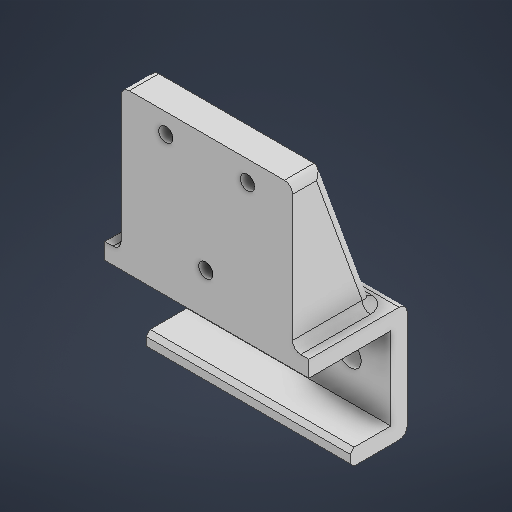
# Autodesk Inventor part: Optical Camera 8020 Bracket
Saved by Autodesk Inventor 2026.2 (Build 302298000, 298)
## iProperties
Created: 2026-02-05
Part Number: Optical Camera 8020 Bracket
Material: Generic
Document SubType Name: Modeling
Designer: mumin
Density: 1 g/cm^3
Appearance: Default
Author: mumin
Autodesk Inventor part; units mm, degrees
ref_plane "YZ Plane" through (0, 0, 0) normal (1, 0, 0) x (0, 1, 0)
ref_plane "XZ Plane" through (0, 0, 0) normal (0, 1, 0) x (-1, 0, 0)
ref_plane "XY Plane" through (0, 0, 0) normal (0, 0, 1) x (1, 0, 0)
sketch "Sketch1" plane through (0, 0, 0) normal (1, 0, 0) x (0, 1, 0)
  line L0 (0, 0) -> (0, -20.1)
  line L1 (0, -20.1) -> (-20.2, -20.1)
  line L2 (-20.2, -20.1) -> (-20.2, -10.1)
  line L3 (-20.2, -10.1) -> (-24.2, -10.1)
  line L4 (-24.2, -10.1) -> (-24.2, -22.1)
  line L5 (-22.2, -24.1) -> (2, -24.1)
  line L6 (4, -22.1) -> (4, 0)
  line L7 (4, 0) -> (0, 0)
  arc A0 (-24.2, -22.1) -> (-22.2, -24.1) centre (-22.2, -22.1) ccw
  arc A1 (2, -24.1) -> (4, -22.1) centre (2, -22.1) ccw
  line L8 (4, 0) -> (39, 0)
  line L9 (39, 0) -> (39, -7.25)
  line L10 (39, -7.25) -> (4, -7.25)
  dimension "d0" = 20.1
  dimension "d1" = 20.2
  dimension "d2" = 10
  dimension "d3" = 4
  dimension "d4" = 4
  dimension "d5" = 4
  dimension "d7" = 35
  dimension "d8" = 7.25
  constraints: 22 end point, 9 perpendicular, 4 point on circle, 4 tangent, 2 centre point, 1 horizontal, 1 point on line, 1 vertical
  measures "d0" distance of L0.start L0.end
  measures "d1" distance of L0.end L1.end
  measures "d2" distance of L1.end L2.end
  measures "d3" distance of L3.end L2.end
  measures "d4" distance between parallel lines of L5 L1
  measures "d5" distance between parallel lines of L0 L6
  measures "d7" distance of L6.end L8.end
  measures "d8" distance of L8.end L9.end
extrude "Beam Clip" add sketch "Sketch1" along normal mid plane 50 contours L7 L6 A1 L5 A0 L4 L3 L2 L1 L0
extrude "Camera Mount Face" add sketch "Sketch1" along normal mid plane 32 contours L8 L9 L10 L6
sketch "Sketch2" plane through (16, 39, -7.25) normal (0, 0, -1) x (-1, 0, 0)
  line L0 (16.0101, -1.1873) -> (16.2932, -34.4018)
  line L1 (32, 0) -> (0, 0) projected
  point P0 (16, -39)
  point P1 (16, 0)
  point P2 (16.2446, -28.7)
  point P3 (6.0422, -5)
  point P4 (26.0415, -4.8296)
  dimension "d14" = 20
  dimension "d38" = 5
  dimension "d39" = 23.7
  constraints: 2 end point, 2 point on line, 1 midpoint, 1 symmetric about line
  measures "d14" diameter of point (6.042, -5) L0
  measures "d38" distance from line of L1 point (6.042, -5)
  measures "d39" vertical distance of point (16.245, -28.7) point (6.042, -5)
hole "Camera Mount Holes" at (-10.0415, 34.1704, -7.25) at (-0.2446, 10.3, -7.25) at (9.9578, 34, -7.25) direction (0, 0, 1) diameter 3.5 end through all
sketch "Sketch3" plane through (16, 0, 0) normal (1, 0, 0) x (0, 0, -1)
  line L0 (7.25, 4) -> (7.25, 39) projected
  line L1 (7.25, 39) -> (19.9087, 4)
  line L2 (22.1, 4) -> (0, 4) projected
  line L3 (0, 39) -> (0, 4) projected
  line L4 (0, 4) -> (0, 39)
  line L5 (0, 39) -> (7.25, 39)
  point P0 (0, 0)
  constraints: 6 end point, 1 perpendicular, 1 point on line, 1 vertical
extrude "Side Rib" add sketch "Sketch3" along normal blind 5
mirror "Rib Mirror" about plane through (0, 0, 0) normal (1, 0, 0) of "Side Rib"
fillet "Rib Edge Fillets" radius 2 12 edges at (21, 4, -9.9544) (18.5, 4, -19.9087) (16, 4, -13.5794) (-18.5, 4, -19.9087) (-16, 4, -13.5794) (-21, 4, -9.9544) (-21, 21.5, -13.5794) (-16, 21.5, -13.5794) (21, 21.5, -13.5794) (16, 21.5, -13.5794) (21, 39, -3.625) (-21, 39, -3.625)
sketch "Sketch4" plane through (25, 2, -24.1) normal (0, 0, -1) x (-1, 0, 0)
  line L0 (50, -22.2) -> (0, -22.2) projected
  line L1 (0, -2) -> (0, -22.2) projected
  line L2 (0, -2) -> (50, -2) projected
  line L3 (50, -22.2) -> (50, -2) projected
  line L4 (0, -24.2) -> (0, 0) projected
  line L5 (0, -12.1) -> (50, -12.1)
  line L6 (25, -2) -> (25, -22.2)
  line L7 (50, -22.2) -> (0, -22.2) projected
  point P0 (25, -2)
  point P1 (10, -12.1)
  point P2 (40, -12.1)
  dimension "d26" = 30
  constraints: 4 end point, 4 midpoint, 2 point on line, 1 symmetric about line
  measures "d26" diameter of point (10, -12.1) L6
hole "8020 Bolt Mount Holes" at (15, -10.1, -24.1) at (-15, -10.1, -24.1) direction (0, 0, 1) diameter 5.5 end through all
chamfer "Chamfer1" distance 1 angle 45 2 edges at (0, -20.2, -10.1) (0, -24.2, -10.1)
body "Solid1"
